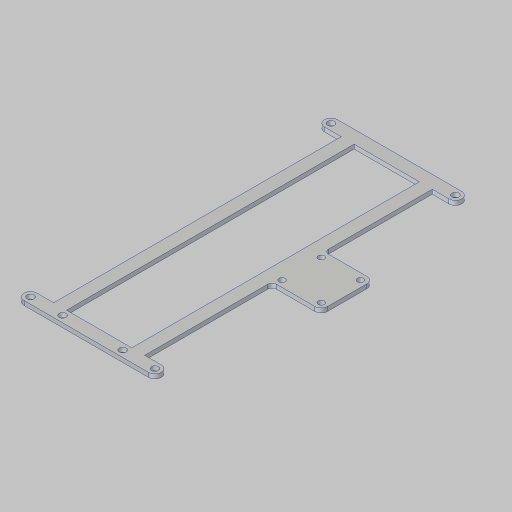
# Autodesk Inventor part: DB1-007
Saved by Autodesk Inventor 2023.5 (Build 275446000, 446)
## iProperties
Created: 2025-01-15
Part Number: DB1-007
Material: Aluminum 6061
Document SubType Name: Modeling
Designer: mavericks
Density: 2.7 g/cm^3
Appearance: Aluminum - Flat
Mass: 54.655 g
Surface Area: 170.066 cm^2
Volume: 20.2426 cm^3
Author: mavericks
Autodesk Inventor part; units mm, degrees
ref_plane "YZ Plane" through (0, 0, 0) normal (1, 0, 0) x (0, 1, 0)
ref_plane "XZ Plane" through (0, 0, 0) normal (0, 1, 0) x (-1, 0, 0)
ref_plane "XY Plane" through (0, 0, 0) normal (0, 0, 1) x (1, 0, 0)
sketch "Sketch1" plane through (0, 0, 0) normal (0, 1, 0) x (-1, 0, 0)
  line L0 (45.974, 111.125) -> (-45.974, 111.125) construction
  line L1 (45.974, 115.8875) -> (-45.974, 115.8875)
  line L2 (-45.974, 106.3625) -> (45.974, 106.3625)
  arc A0 (45.974, 106.3625) -> (45.974, 115.8875) centre (45.974, 111.125) ccw
  arc A1 (-45.974, 115.8875) -> (-45.974, 106.3625) centre (-45.974, 111.125) ccw
  line L3 (0, 111.125) -> (0, -111.125) construction
  line L4 (45.974, -111.125) -> (-45.974, -111.125) construction
  line L5 (45.974, -115.8875) -> (-45.974, -115.8875)
  line L6 (-45.974, -106.3625) -> (45.974, -106.3625) construction
  arc A2 (45.974, -115.8875) -> (45.974, -106.3625) centre (45.974, -111.125) ccw
  arc A3 (-45.974, -106.3625) -> (-45.974, -115.8875) centre (-45.974, -111.125) ccw
  line L7 (24.13, 106.3625) -> (24.13, -106.3625)
  line L8 (-24.13, 106.3625) -> (-24.13, -106.3625) construction
  line L9 (24.13, 0) -> (-24.13, 0) construction
  line L10 (33.655, 106.3625) -> (33.655, -106.3625)
  line L11 (-33.655, 106.3625) -> (-33.655, -106.3625)
  line L12 (45.974, -106.3625) -> (33.655, -106.3625)
  line L13 (-24.13, -106.3625) -> (24.13, -106.3625)
  line L14 (-24.13, -106.3625) -> (-24.13, 106.3625)
  line L15 (-33.655, -106.3625) -> (-45.974, -106.3625)
  line L16 (14.478, 14.478) -> (-14.478, -14.478) construction
  circle A4 centre (14.478, 14.478) radius 4.7625 construction
  circle A5 centre (-14.478, -14.478) radius 4.7625 construction
  line L17 (11.1788, 17.9127) -> (24.13, 30.353)
  line L18 (11.1788, 11.0433) -> (24.13, -1.397)
  line L19 (-11.1788, -17.9127) -> (-24.13, -30.353)
  line L20 (-11.1788, -11.0433) -> (-24.13, 1.397)
  arc A6 (11.1788, 17.9127) -> (11.1788, 11.0433) centre (14.478, 14.478) ccw
  arc A7 (-11.1788, -17.9127) -> (-11.1788, -11.0433) centre (-14.478, -14.478) ccw
  point P0 (0, 0)
  point P1 (0, 0)
  point P2 (0, 0)
  point P3 (-33.655, 106.3625)
  point P4 (33.655, 106.3625)
  point P5 (0, 0)
  dimension "d0" = 9.525
  dimension "d1" = 91.948
  dimension "d2" = 222.25
  dimension "d4" = 9.525
  dimension "d5" = 48.26
  dimension "d6" = 9.525
  dimension "d7" = 9.525
  dimension "d33" = 28.956
  dimension "d34" = 28.956
  dimension "d35" = 9.525
  dimension "d36" = 9.525
  dimension "d37" = 15.875
  dimension "d38" = 15.875
  dimension "d39" = 15.875
  dimension "d40" = 15.875
  constraints: 46 end point, 16 point on circle, 12 tangent, 10 point on line, 8 centre point, 8 coincident, 7 midpoint, 5 parallel, 4 collinear, 3 vertical alignment, 2 horizontal, 1 perpendicular, 1 vertical
  measures "d0" diameter of A1
  measures "d1" distance of L0.end L0.start
  measures "d2" distance of L3.start L3.end
  measures "d4" distance of L5.end L6.start
  measures "d5" distance between parallel lines of L8 L7
  measures "d6" distance between parallel lines of L7 L10
  measures "d7" distance between parallel lines of L8 L11
  measures "d33" horizontal distance of L16.end L16.start
  measures "d34" horizontal distance of L16.start L16.end
  measures "d35" diameter of A4
  measures "d36" diameter of A5
  measures "d37" vertical distance of L17.end A4.centre
  measures "d38" vertical distance of L18.end A4.centre
  measures "d39" vertical distance of A5.centre L20.end
  measures "d40" vertical distance of L19.end A5.centre
extrude "Extrusion1" add sketch "Sketch1" along normal blind 3.175 contours A0 L2 A1 L1 | L10 L12 A2 L5 A3 L15 L11 L2 L14 L13 L7
sketch "Sketch2" plane through (0, 3.175, 0) normal (0, 1, 0) x (1, 0, 0)
  line L0 (-33.655, -106.3625) -> (-45.974, -106.3625) construction
  arc A0 (-45.974, -106.3625) -> (-45.974, -115.8875) centre (-45.974, -111.125) ccw construction
  line L1 (-45.974, -115.8875) -> (45.974, -115.8875) construction
  arc A1 (45.974, -115.8875) -> (45.974, -106.3625) centre (45.974, -111.125) ccw construction
  line L2 (-24.13, -106.3625) -> (-24.13, 106.3625) projected
  line L3 (-24.13, 106.3625) -> (24.13, 106.3625) projected
  line L4 (24.13, 106.3625) -> (24.13, -106.3625) projected
  line L5 (24.13, -106.3625) -> (-24.13, -106.3625) projected
  line L6 (45.974, -106.3625) -> (33.655, -106.3625) projected
  line L7 (33.655, -106.3625) -> (33.655, 106.3625) projected
  line L8 (33.655, 106.3625) -> (45.974, 106.3625) projected
  arc A2 (45.974, 106.3625) -> (45.974, 115.8875) centre (45.974, 111.125) ccw projected
  line L9 (45.974, 115.8875) -> (-45.974, 115.8875) projected
  arc A3 (-45.974, 115.8875) -> (-45.974, 106.3625) centre (-45.974, 111.125) ccw projected
  line L10 (-45.974, 106.3625) -> (-33.655, 106.3625) projected
  line L11 (-33.655, 106.3625) -> (-33.655, -106.3625) projected
  point P0 (0, 0)
  point P1 (45.974, 111.125)
  point P2 (-45.974, 111.125)
  point P3 (-14.478, 71.0565)
  point P4 (14.478, 100.0125)
  constraints: 2 coincident
hole "Hole1" at (-45.974, 3.175, 111.125) at (45.974, 3.175, 111.125) at (45.974, 3.175, -111.125) at (-45.974, 3.175, -111.125) direction (0, -1, 0) diameter 5.1054 end through all clearance for "Flat Head Machine Screw (82)" size "#10" standard "Ansi Unified Screw Threads"
sketch "Sketch3" plane through (0, 3.175, 0) normal (0, 1, 0) x (1, 0, 0)
  circle A0 centre (45.974, 111.125) radius 2.5527 construction
  circle A1 centre (-45.974, -111.125) radius 2.5527 construction
  circle A2 centre (45.974, -111.125) radius 2.5527 construction
  circle A3 centre (-45.974, 111.125) radius 2.5527 construction
  line L0 (-24.13, -106.3625) -> (24.13, -106.3625) construction
  line L1 (24.13, -106.3625) -> (24.13, 106.3625) construction
  line L2 (24.13, 106.3625) -> (-24.13, 106.3625) construction
  line L3 (-24.13, 106.3625) -> (-24.13, -106.3625) construction
  line L4 (-33.655, -106.3625) -> (-33.655, 106.3625) construction
  line L5 (-33.655, 106.3625) -> (-45.974, 106.3625) construction
  arc A4 (-45.974, 115.8875) -> (-45.974, 106.3625) centre (-45.974, 111.125) ccw construction
  line L6 (-45.974, 115.8875) -> (45.974, 115.8875) construction
  arc A5 (45.974, 106.3625) -> (45.974, 115.8875) centre (45.974, 111.125) ccw construction
  line L7 (45.974, 106.3625) -> (33.655, 106.3625) construction
  line L8 (33.655, 106.3625) -> (33.655, -106.3625) construction
  line L9 (33.655, -106.3625) -> (45.974, -106.3625) construction
  arc A6 (45.974, -115.8875) -> (45.974, -106.3625) centre (45.974, -111.125) ccw construction
  line L10 (45.974, -115.8875) -> (-45.974, -115.8875) construction
  arc A7 (-45.974, -106.3625) -> (-45.974, -115.8875) centre (-45.974, -111.125) ccw construction
  line L11 (-45.974, -106.3625) -> (-33.655, -106.3625) construction
  line L12 (65.278, -7.366) -> (36.322, 21.59) construction
  circle A8 centre (65.278, -7.366) radius 4.7625 construction
  circle A9 centre (36.322, 21.59) radius 4.7625 construction
  line L13 (33.655, -106.3625) -> (33.655, 106.3625) construction
  circle A10 centre (36.322, -7.366) radius 4.7625 construction
  circle A11 centre (65.278, 21.59) radius 4.7625 construction
  line L14 (33.655, -12.1285) -> (65.278, -12.1285)
  line L15 (70.0405, -7.366) -> (70.0405, 21.59)
  line L16 (65.278, 26.3525) -> (33.655, 26.3525)
  arc A12 (65.278, -12.1285) -> (70.0405, -7.366) centre (65.278, -7.366) ccw
  arc A13 (70.0405, 21.59) -> (65.278, 26.3525) centre (65.278, 21.59) ccw
  line L17 (33.655, -12.1285) -> (33.655, 26.3525)
  point P0 (0, 0)
  point P1 (50.8, 7.112)
  dimension "d48" = 31.623
  dimension "d50" = 28.956
  dimension "d51" = 9.525
  dimension "d66" = 7.112
  dimension "d67" = 28.956
  constraints: 10 end point, 8 point on circle, 6 centre point, 6 coincident, 4 tangent, 3 equal radius, 2 horizontal alignment, 2 perpendicular, 2 point on line, 2 vertical alignment, 1 collinear, 1 midpoint
  measures "d48" distance from line of L8 L12.start
  measures "d50" horizontal distance of L12.end L12.start
  measures "d51" diameter of A8
  measures "d66" vertical distance of point (0, 0) point (50.8, 7.112)
  measures "d67" distance of A11.centre A9.centre
extrude "Extrusion2" add sketch "Sketch3" against normal blind 3.175
fillet "Fillet2" radius 3.302 2 edges at (33.655, 1.5875, 12.1285) (33.655, 1.5875, -26.3525)
hole "Hole4" at (65.278, 3.175, 7.366) at (36.322, 3.175, -21.59) at (36.322, 3.175, 7.366) at (65.278, 3.175, -21.59) direction (0, -1, 0) diameter 4.4958 end through all clearance for "Flat Head Machine Screw (82)" size "#8" standard "Ansi Unified Screw Threads"
sketch "Sketch4" plane through (0, 3.175, 0) normal (0, 1, 0) x (1, 0, 0)
  line L0 (22.225, -111.125) -> (-22.225, -111.125) construction
  circle A0 centre (36.322, -7.366) radius 2.2479 construction
  circle A1 centre (65.278, -7.366) radius 2.2479 construction
  circle A2 centre (36.322, 21.59) radius 2.2479 construction
  circle A3 centre (65.278, 21.59) radius 2.2479 construction
  circle A4 centre (45.974, 111.125) radius 2.5527 construction
  circle A5 centre (-45.974, -111.125) radius 2.5527 construction
  circle A6 centre (45.974, -111.125) radius 2.5527 construction
  circle A7 centre (-45.974, 111.125) radius 2.5527 construction
  line L1 (-24.13, -106.3625) -> (-24.13, 106.3625) construction
  line L2 (-24.13, 106.3625) -> (24.13, 106.3625) construction
  line L3 (24.13, 106.3625) -> (24.13, -106.3625) construction
  line L4 (24.13, -106.3625) -> (-24.13, -106.3625) construction
  line L5 (-33.655, -106.3625) -> (-45.974, -106.3625) construction
  arc A8 (-45.974, -106.3625) -> (-45.974, -115.8875) centre (-45.974, -111.125) ccw construction
  line L6 (-45.974, -115.8875) -> (45.974, -115.8875) construction
  arc A9 (45.974, -115.8875) -> (45.974, -106.3625) centre (45.974, -111.125) ccw construction
  line L7 (45.974, -106.3625) -> (33.655, -106.3625) construction
  line L8 (33.655, -106.3625) -> (33.655, -15.4305) construction
  arc A10 (36.957, -12.1285) -> (33.655, -15.4305) centre (36.957, -15.4305) ccw construction
  line L9 (36.957, -12.1285) -> (65.278, -12.1285) construction
  arc A11 (65.278, -12.1285) -> (70.0405, -7.366) centre (65.278, -7.366) ccw construction
  line L10 (70.0405, -7.366) -> (70.0405, 21.59) construction
  arc A12 (70.0405, 21.59) -> (65.278, 26.3525) centre (65.278, 21.59) ccw construction
  line L11 (65.278, 26.3525) -> (36.957, 26.3525) construction
  arc A13 (33.655, 29.6545) -> (36.957, 26.3525) centre (36.957, 29.6545) ccw construction
  line L12 (33.655, 29.6545) -> (33.655, 106.3625) construction
  line L13 (33.655, 106.3625) -> (45.974, 106.3625) construction
  arc A14 (45.974, 106.3625) -> (45.974, 115.8875) centre (45.974, 111.125) ccw construction
  line L14 (45.974, 115.8875) -> (-45.974, 115.8875) construction
  arc A15 (-45.974, 115.8875) -> (-45.974, 106.3625) centre (-45.974, 111.125) ccw construction
  line L15 (-45.974, 106.3625) -> (-33.655, 106.3625) construction
  line L16 (-33.655, 106.3625) -> (-33.655, -106.3625) construction
  point P0 (0, 0)
  point P1 (0, -111.125)
  point P2 (0, -115.8875)
  dimension "d68" = 44.45
  constraints: 2 end point, 2 horizontal alignment, 2 midpoint, 1 horizontal, 1 vertical alignment
  measures "d68" distance of L0.start L0.end
hole "Hole5" at (22.225, 3.175, 111.125) at (-22.225, 3.175, 111.125) direction (0, -1, 0) diameter 5.1054 end through all clearance for "Flat Head Machine Screw (82)" size "#10" standard "Ansi Unified Screw Threads"
equation "\"d4\" = d0"
equation "\"d6\" = d7"
equation "\"d38\" = d37"
equation "\"d39\" = d37"
equation "\"d40\" = d39"
body "Solid1"
